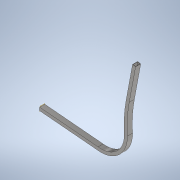
# Autodesk Inventor part: Asiento nuevo
Saved by Autodesk Inventor 2021 (Build 250183000, 183)
## iProperties
Created: 2014-11-01
Part Number: Asiento nuevo
Material: Acero, suave
Document SubType Name: Modeling
Designer: Yeison
Density: 7.85 g/cm^3
Appearance: Semipulido
Sending System: SolidWorks 2014
Last Author: JFGC
Last Saved: 2014-11-06
Author: Yeison
Autodesk Inventor part; units mm, degrees
ref_plane "YZ Plane" through (0, 0, 0) normal (1, 0, 0) x (0, 1, 0)
ref_plane "XZ Plane" through (0, 0, 0) normal (0, 1, 0) x (-1, 0, 0)
ref_plane "XY Plane" through (0, 0, 0) normal (0, 0, 1) x (1, 0, 0)
sketch "Boceto8" plane through (0, 0, 0) normal (0, 0, 1) x (1, 0, 0)
  line L0 (94.4495, 6.2065) -> (380.596, -19.1326)
  arc A0 (380.596, -19.1326) -> (517.3175, 105.3044) centre (396.805, 100.386) ccw
  arc A1 (526.695, 255.3458) -> (517.3175, 105.3044) centre (1130.7459, 142.2789) ccw
  line L1 (526.695, 255.3458) -> (557.7708, 421.3657)
  point P0 (0, 0)
  constraints: 4 end point, 4 point on circle, 2 centre point
ref_plane "Plano transversal al perfil" through (94.4495, 6.2065, 0) normal (0.9961021, -0.0882078, 0) x (0.0882078, 0.9961021, 0)
sketch "Boceto9" plane through (94.4495, 6.2065, 0) normal (0.9961021, -0.0882078, 0) x (0.0882078, 0.9961021, 0)
  line L0 (7.5, 12.5084) -> (-7.5, 12.5084)
  line L1 (-7.5, 12.5084) -> (-7.5, -12.4916)
  line L2 (-7.5, -12.4916) -> (7.5, -12.4916)
  line L3 (7.5, -12.4916) -> (7.5, 12.5084)
  line L4 (0, 0.0084) -> (0, -12.4916)
  line L5 (6, 11.0084) -> (-6, 11.0084)
  line L6 (-6, 11.0084) -> (-6, -10.9916)
  line L7 (-6, -10.9916) -> (6, -10.9916)
  line L8 (6, -10.9916) -> (6, 11.0084)
  point P0 (-14.5135, 0)
  dimension "h_a" = 15
  dimension "w_a" = 25
  dimension "w_a2" = 12.5
  dimension "t_a" = 1.5
  constraints: 18 end point, 4 parallel, 2 perpendicular, 1 horizontal, 1 midpoint, 1 vertical, 3 other
  measures "h_a" distance of L2.end L1.end
  measures "w_a" distance of L1.end L0.end
  measures "w_a2" distance of L4.start L4.end
  measures "t_a" distance between parallel lines of L3 L8
sweep "Barrido2" add profiles "Boceto9" path "Boceto8"
equation "\"w_a2\" = 0.5 * w_a"
